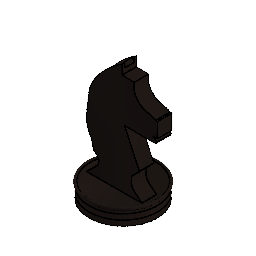
Knight Piece (Autodesk Fusion 360 design; units mm, degrees)
Autodesk Fusion 360 part; units mm, degrees
sketch "Sketch13" plane through (0, 0, 0) normal (0, 1, 0) x (1, 0, 0)
sketch "Sketch14" plane through (0, 0, 0) normal (0, 1, 0) x (1, 0, 0)
  line L0 (0, 0) -> (-2.5, 0)
  line L1 (-2.5, 0) -> (-2.5, -0.4)
  spline S0 degree 5 poles (-2.5, -0.4) (-2.4983, -0.404) (-2.4944, -0.412) (-2.487, -0.424) (-2.4743, -0.44) (-2.4536, -0.46) (-2.4286, -0.48) (-2.4004, -0.5) (-2.3706, -0.52) (-2.3423, -0.54) (-2.3186, -0.56) (-2.3028, -0.58) (-2.2972, -0.6) (-2.3028, -0.62) (-2.3186, -0.64) (-2.3423, -0.66) (-2.3706, -0.68) (-2.4004, -0.7) (-2.4286, -0.72) (-2.4536, -0.74) (-2.4743, -0.76) (-2.487, -0.776) (-2.4944, -0.788) (-2.4983, -0.796) (-2.5, -0.8) knots 0 0 0 0 0 0 0.05 0.1 0.15 0.2 0.25 0.3 0.35 0.4 0.45 0.5 0.55 0.6 0.65 0.7 0.75 0.8 0.85 0.9 0.95 1 1 1 1 1 1
  line L2 (-2.5, -0.8) -> (-2.5, -0.9)
  line L3 (-2.5, -0.9) -> (-2.5, -1)
  line L4 (-2.4, -1.1) -> (0, -1.1)
  line L5 (0, -1.1) -> (0, 0)
  arc A0 (-2.5, -1) -> (-2.4, -1.1) centre (-2.5, -1.1) ccw
  line L6 (-2.5133, -0.3689) -> (-2.4867, -0.4311)
  line L7 (-2.4867, -0.7689) -> (-2.5133, -0.8311)
  spline S1 degree 5 poles (-1.2, -1.1) (-1.1897, -1.1117) (-1.1694, -1.1344) (-1.1395, -1.1669) (-1.1008, -1.2068) (-1.0544, -1.2515) (-1.0094, -1.2921) (-0.9649, -1.3306) (-0.9195, -1.3707) (-0.8716, -1.4164) (-0.8213, -1.4712) (-0.7706, -1.5362) (-0.7252, -1.6089) (-0.6936, -1.6836) (-0.6835, -1.754) (-0.6995, -1.8152) (-0.74, -1.8657) (-0.7957, -1.909) (-0.8543, -1.9511) (-0.9042, -1.9981) (-0.9384, -2.0544) (-0.9589, -2.1204) (-0.973, -2.1939) (-0.9895, -2.272) (-1.0157, -2.3519) (-1.0537, -2.4334) (-1.0996, -2.5179) (-1.1474, -2.608) (-1.1896, -2.7065) (-1.2202, -2.815) (-1.2365, -2.9337) (-1.2395, -3.0608) (-1.2322, -3.1933) (-1.219, -3.3279) (-1.2039, -3.4615) (-1.1902, -3.5915) (-1.1783, -3.7171) (-1.1669, -3.8386) (-1.1532, -3.9571) (-1.1338, -4.0741) (-1.1054, -4.1911) (-1.0657, -4.309) (-1.014, -4.4275) (-0.9511, -4.5459) (-0.8786, -4.6627) (-0.7987, -4.7763) (-0.714, -4.8852) (-0.6266, -4.9881) (-0.5383, -5.0843) (-0.4503, -5.1738) (-0.3633, -5.257) (-0.2776, -5.3342) (-0.1936, -5.4062) (-0.1113, -5.4735) (-0.0307, -5.5364) (0.0481, -5.5952) (0.1098, -5.6391) (0.1552, -5.6702) (0.1851, -5.6902) (0.2, -5.7) knots 0 0 0 0 0 0 0.018182 0.036364 0.054545 0.072727 0.090909 0.109091 0.127273 0.145455 0.163636 0.181818 0.2 0.218182 0.236364 0.254545 0.272727 0.290909 0.309091 0.327273 0.345455 0.363636 0.381818 0.4 0.418182 0.436364 0.454545 0.472727 0.490909 0.509091 0.527273 0.545455 0.563636 0.581818 0.6 0.618182 0.636364 0.654545 0.672727 0.690909 0.709091 0.727273 0.745455 0.763636 0.781818 0.8 0.818182 0.836364 0.854545 0.872727 0.890909 0.909091 0.927273 0.945455 0.963636 0.981818 1 1 1 1 1 1
  line L8 (0.2, -5.7) -> (0.2, -5.3)
  line L9 (0.2, -5.3) -> (0.7, -5.3)
  spline S2 degree 5 poles (0.7, -5.3) (0.6977, -5.2852) (0.6936, -5.2561) (0.6888, -5.2143) (0.6851, -5.1621) (0.685, -5.1028) (0.6895, -5.0493) (0.6984, -5.0009) (0.7118, -4.9568) (0.7293, -4.9155) (0.7507, -4.8753) (0.7758, -4.8347) (0.8046, -4.7926) (0.8369, -4.7492) (0.8733, -4.7057) (0.9139, -4.6637) (0.9591, -4.6255) (1.0091, -4.5925) (1.0634, -4.5656) (1.1213, -4.5443) (1.1819, -4.5272) (1.2439, -4.5127) (1.3062, -4.4988) (1.368, -4.484) (1.4285, -4.4673) (1.4876, -4.4479) (1.5334, -4.4302) (1.567, -4.4156) (1.5891, -4.4053) (1.6, -4.4) knots 0 0 0 0 0 0 0.04 0.08 0.12 0.16 0.2 0.24 0.28 0.32 0.36 0.4 0.44 0.48 0.52 0.56 0.6 0.64 0.68 0.72 0.76 0.8 0.84 0.88 0.92 0.96 1 1 1 1 1 1
  arc A1 (1.6727, -4.4) -> (1.6, -4.4) centre (1.6363, -4.475) ccw
  line L10 (1.6727, -4.4) -> (1.6727, -3.7734)
  line L11 (1.6727, -3.7734) -> (1.5, -3.7734)
  line L12 (1.5, -3.7734) -> (1.6727, -3.6602)
  line L13 (1.6727, -3.6602) -> (1.6037, -3.555)
  line L14 (1.6037, -3.555) -> (0.3262, -3.555)
  line L15 (0.3262, -3.555) -> (0.9649, -2.2384)
  line L16 (0.9649, -2.2384) -> (0.6455, -1.8916)
  spline S3 degree 5 poles (0.6455, -1.8916) (0.6462, -1.887) (0.6472, -1.8774) (0.6484, -1.8617) (0.649, -1.8385) (0.6483, -1.8055) (0.6467, -1.7685) (0.6449, -1.7279) (0.6447, -1.6839) (0.6481, -1.6373) (0.6578, -1.589) (0.6758, -1.5398) (0.7034, -1.4909) (0.7406, -1.443) (0.7856, -1.3971) (0.8355, -1.3537) (0.887, -1.3135) (0.9365, -1.2769) (0.981, -1.2442) (1.0187, -1.2156) (1.0484, -1.1911) (1.0656, -1.1748) (1.0746, -1.1645) (1.079, -1.1583) (1.0807, -1.1555) knots 0 0 0 0 0 0 0.05 0.1 0.15 0.2 0.25 0.3 0.35 0.4 0.45 0.5 0.55 0.6 0.65 0.7 0.75 0.8 0.85 0.9 0.95 1 1 1 1 1 1
  line L17 (-1.2, -1.1) -> (1.0807, -1.1555)
  point P0 (-2.4, -0.5)
  point P1 (-2.3, -0.6)
  point P2 (-2.4, -0.7)
  point P3 (-1, -1.3)
  point P4 (-0.8, -1.5)
  point P5 (-0.7, -1.8)
  point P6 (-0.9, -2)
  point P7 (-1, -2.3)
  point P8 (-1.2, -2.7505)
  point P9 (-1.2, -3.5)
  point P10 (-1.1, -4.2)
  point P11 (-0.7, -4.9)
  point P12 (-0.2, -5.4)
  point P13 (0.7, -5)
  point P14 (0.8, -4.8)
  point P15 (1, -4.6)
  point P16 (1.3, -4.5)
  point P17 (0.6455, -1.7369)
  point P18 (0.7, -1.5)
  point P19 (0.942, -1.2728)
  constraint coincident L0.start L5.end
  constraint horizontal L0
  constraint perpendicular L0 L1
  constraint vertical L2
  constraint parallel L2 L3
  constraint coincident A0.centre L4
  constraint horizontal L4
  constraint perpendicular L0 L5
  constraint midpoint L1.end L6
  constraint midpoint S0.end L7
  constraint vertical L8
  constraint perpendicular L8 L9
  constraint tangent S2 A1
  constraint vertical L10
  constraint perpendicular L10 L11
  constraint perpendicular L12 L13
  constraint perpendicular L10 L14
revolve "Revolve2" add sketch "Sketch14" angle 360 about axis through (0, 0, 1.1) along (0, 0, -1) contours L0 L1 S0 L2 L3 L4 L5 A0 makes body 1
extrude "Extrude1" add sketch "Sketch14" along normal blind 0.3 and the other way blind 0.3 separate body contours S1 L8 L9 S2 A1 L10 L11 L12 L13 L14 L15 L16 S3 L17 makes body 2
scale "Scale1" factor 0.75 about (-2.5, 0, 1) bodies 1
move_body "Move1" bodies 1 to x (1, 0, 0) y (0, 1, 0) z (0, 0, 1) at (0.2643, 0.1459, -0.1184)
move_body "Move2" bodies 1 to x (1, 0, 0) y (0, 1, 0) z (0, 0, 1) at (0.3032, 0, -0.1582)
move_body "Move3" bodies 2 to x (0.999848, 0, -0.017452) y (0, 1, 0) z (0.017452, 0, 0.999848) at (0.0447, 0, -0.2578)
scale "Scale2" factor 0.75 about (-1.8575, 0.1459, 0.7984) bodies 1
move_body "Move4" bodies 1 to x (1, 0, 0) y (0, 1, 0) z (0, 0, 1) at (0.4411, 0, -0.1697)
move_body "Move5" bodies 2 to x (1, 0, 0) y (0, 1, 0) z (0, 0, 1) at (0, 0, -0.2036)
ref_plane "WorkPlane6" through (0.3441, 0, 5.2343) normal (-0.5, 0, 0.866025) x (0, -1, 0)
sketch "Sketch15" plane through (0.3441, 0, 5.2343) normal (-0.5, 0, 0.866025) x (0, -1, 0)
  line L0 (-0.2, 0.1) -> (0.2, 0.1)
  line L1 (0.2, 0.1) -> (0.2, -0.1)
  line L2 (0.2, -0.1) -> (-0.2, -0.1)
  line L3 (-0.2, -0.1) -> (-0.2, 0.1)
  constraint horizontal L0
  constraint vertical L1
  constraint horizontal L2
  constraint vertical L3
extrude "Extrude2" cut sketch "Sketch15" along normal blind 0 and the other way blind 0.2 bodies 2
copy_body "CopyPasteBodies1" bodies 2 1 makes body 3 makes body 4
copy_body "CopyPasteBodies2" bodies 2 4 3 1 makes body 5 makes body 6 makes body 7 makes body 8
sketch "Sketch1" plane through (0, 0, 0) normal (0, 1, 0) x (1, 0, 0)
  line L0 (0, 0) -> (-10, 0)
  spline S0 degree 5 poles (-10.1038, -4) (-10.0793, -3.9976) (-10.027, -3.9957) (-9.9387, -4.0008) (-9.8011, -4.024) (-9.597, -4.0804) (-9.365, -4.1644) (-9.1134, -4.2755) (-8.8577, -4.4126) (-8.6204, -4.5734) (-8.4266, -4.7547) (-8.2995, -4.9522) (-8.2566, -5.1607) (-8.3047, -5.3736) (-8.4363, -5.5836) (-8.6338, -5.7824) (-8.8739, -5.9623) (-9.1319, -6.1159) (-9.3856, -6.2376) (-9.6199, -6.3237) (-9.8262, -6.3727) (-9.9658, -6.3819) (-10.0558, -6.3719) (-10.1092, -6.3578) (-10.1343, -6.3489) knots 0 0 0 0 0 0 0.05 0.1 0.15 0.2 0.25 0.3 0.35 0.4 0.45 0.5 0.55 0.6 0.65 0.7 0.75 0.8 0.85 0.9 0.95 1 1 1 1 1 1
  line L1 (-9.2933, -11.9206) -> (0, -11.9206)
  line L2 (0, -11.9206) -> (0, 0)
  arc A0 (-10.0331, -9.8399) -> (-9.2933, -11.9206) centre (-10, -11) ccw
  line L3 (-10.1343, -6.3489) -> (-10.1343, -8.5)
  line L4 (-10.1343, -8.5) -> (-10.5, -8.5)
  line L5 (-10.5, -8.5) -> (-10.0331, -8.9783)
  line L6 (-10.0331, -8.9783) -> (-10.0331, -9.8399)
  line L7 (-10, 0) -> (-10, -2.0122)
  line L8 (-10, -2.0122) -> (-10.5365, -2.0122)
  line L9 (-10.5365, -2.0122) -> (-10.1038, -2.4439)
  line L10 (-10.1038, -2.4439) -> (-10.1038, -3)
  line L11 (-10.1038, -3) -> (-10.1038, -4)
  point P0 (-9.1786, -4.2503)
  point P1 (-8.2792, -5.1497)
  point P2 (-9.1974, -6.1428)
  constraint coincident L0.start L2.end
  constraint horizontal L0
  constraint horizontal L1
  constraint perpendicular L0 L2
  constraint vertical L3
  constraint perpendicular L3 L4
  constraint perpendicular L4 L6
  constraint perpendicular L0 L7
  constraint perpendicular L7 L8
  constraint perpendicular L8 L10
  constraint perpendicular L8 L11
sketch "Sketch12" plane through (-5.6756, 0, 6.2168) normal (0, 1, 0) x (1, 0, 0)
revolve "Revolve1" [suppressed]
sketch "Sketch2" plane through (0, 0, 11.9206) normal (0, 0, 1) x (-1, 0, 0)
  circle A0 centre (0, 0) radius 9.2933
  ellipse E0 centre (0, 0) end of major axis (-6.6057, 0) minor radius 3.1539
  line L0 (6.6057, 0) -> (-6.6057, 0)
  line L1 (0, 3.1539) -> (0, -3.1539)
  constraint coincident A0.centre E0.centre
  constraint horizontal L0
  constraint coincident E0 L0.start
  constraint coincident E0 L0.end
  constraint coincident E0 L1.start
  constraint coincident E0 L1.end
sketch "Sketch3" plane through (0, 0, 11.9206) normal (0, 0, 1) x (1, 0, 0)
sketch "Sketch4" plane through (0, 0, 11.9206) normal (0, 0, 1) x (-1, 0, 0)
ref_plane "WorkPlane2" through (0, 0, 26.9206) normal (0, 0, 1) x (-1, 0, 0)
sketch "Sketch5" plane through (0, 0, 26.9206) normal (0, 0, 1) x (1, 0, 0)
sketch "Sketch6" plane through (0, 0, 26.9206) normal (-0.258819, 0, 0.965926) x (0, -1, 0)
sketch "Sketch7" plane through (0, 0, 26.9206) normal (0, 0, 1) x (1, 0, 0)
ref_plane "WorkPlane4" through (0, 0, 26.9206) normal (-0.173648, 0, 0.984808) x (0, -1, 0)
sketch "Sketch8" plane through (0, 0, 26.9206) normal (-0.173648, 0, 0.984808) x (0, -1, 0)
sketch "Sketch9" plane through (0, 0, 26.9206) normal (0, 0, 1) x (1, 0, 0)
ref_plane "WorkPlane5" through (0, 1, 26.9206) normal (-0.173648, 0, 0.984808) x (0, -1, 0)
sketch "Sketch10" plane through (0, 0, 0) normal (1, 0, 0) x (0, 1, 0)
sketch "Sketch11" plane through (0, 1, 26.9206) normal (-0.173648, 0, 0.984808) x (0, -1, 0)
  curve E0
  line L0 (-0.4345, -6.4605, -1.4371) -> (-0.4345, 6.9495, -1.4371)
  line L1 (2.5673, 0.2445, -1.4518) -> (-3.4363, 0.2445, -1.4223)
  dimension "d7" = 13.41
loft "Loft1" [suppressed]
delete_face "DeleteFace1" [suppressed]
